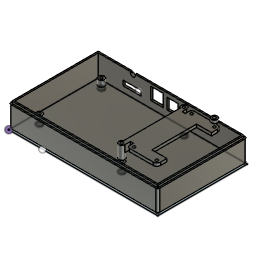
newSandProjectBox (Autodesk Fusion 360 design; units mm, degrees)
Autodesk Fusion 360 part; units mm, degrees
sketch "base " plane through (0, 0, 0) normal (0, 0, 1) x (1, 0, 0)
  line L0 (0, 0) -> (150, 0)
  line L1 (150, 0) -> (150, 90)
  line L2 (150, 90) -> (0, 90)
  line L3 (0, 90) -> (0, 0)
  circle A0 centre (10.5, 82.8) radius 3
  circle A1 centre (93.5, 82.8) radius 3
  circle A2 centre (93.5, 20.3) radius 3
  circle A3 centre (10.5, 20.3) radius 3
  point P0 (34, 0)
  point P1 (31.6409, 99.4995)
  dimension "d1" = 150
  dimension "d2" = 90
  dimension "d5" = 83
  dimension "d6" = 62.5
  dimension "d13" = 6
  dimension "d42" = 7.2
  dimension "d43" = 10.5
  constraint horizontal L0
  constraint vertical L1
  constraint horizontal L2
  constraint vertical L3
  constraint coincident L0.start L3.end
  measures "d1" distance of L0.start L0.end
  measures "d2" distance of L0.start L2.end
  measures "d13" diameter of A3
  measures "d42" distance of L2 A1.centre
  measures "d43" distance of L3 A3.centre
extrude "Extrude1" add sketch "base " along normal blind 25 contours L0 L1 L2 L3 | A0 | A1 | A2 | A3 makes body 1
shell "Shell1" thickness 3 removed faces 1 at (50, 60, 25) on bodies 1
sketch "back" plane through (0, 90, 0) normal (0, 1, 0) x (-1, 0, 0)
  line L0 (-150, 0) -> (0, 0)
  line L1 (0, 0) -> (0, 25)
  line L2 (0, 25) -> (-150, 25)
  line L3 (-150, 25) -> (-150, 0)
  circle A0 centre (-38, 24) radius 2.5
  line L4 (-28, 12.8) -> (-46, 12.8)
  line L5 (-56, 22.5) -> (-56, 10)
  line L6 (0, 25) -> (-123.61, 25)
  line L7 (-46, 12.8) -> (-46, 8.8)
  line L8 (-68.5, 22.5) -> (-56, 22.5)
  line L9 (-72.39, 21) -> (-72.39, 10)
  line L10 (-28, 8.8) -> (-28, 12.8)
  line L11 (-83.39, 10) -> (-83.39, 21)
  line L12 (-68.5, 10) -> (-68.5, 22.5)
  line L13 (-72.39, 10) -> (-83.39, 10)
  line L14 (-83.39, 21) -> (-72.39, 21)
  line L15 (-56, 10) -> (-68.5, 10)
  line L16 (-46, 8.8) -> (-28, 8.8)
  point P0 (0, 25)
  point P1 (-96, 0)
  point P2 (-96, 0)
  dimension "d25" = 12.5
  dimension "d26" = 12.5
  dimension "d27" = 11
  dimension "d28" = 11
  dimension "d34" = 18
  dimension "d35" = 4
  dimension "d37" = 5
  dimension "d107" = 28
  dimension "d108" = 56
  dimension "d109" = 72.39
  constraint horizontal L8
  constraint vertical L5
  constraint horizontal L15
  constraint vertical L12
  constraint horizontal L14
  constraint vertical L9
  constraint horizontal L13
  constraint vertical L11
  constraint coincident P2 P1
  constraint vertical L7
  constraint horizontal L16
  constraint vertical L10
  constraint perpendicular L4 L7
  measures "d25" distance of L8.start L5.start
  measures "d26" distance of L8.start L12.start
  measures "d27" distance of L11.end L9.start
  measures "d28" distance of L11.start L11.end
  measures "d34" distance of L4.end L4.start
  measures "d35" distance of L4.start L10.start
  measures "d37" diameter of A0
  measures "d107" distance of L1 L10
  measures "d108" distance of L1 L5
  measures "d109" distance of L1 L9
extrude "Extrude2" cut sketch "back" against normal blind 10 contours L2 A0 L6 | L4 L7 L10 L16 | L5 L8 L12 L15 | L9 L11 L13 L14 picked at (-38.7711, 24.4201) bodies 1
extrude "Extrude3" add sketch "base " along normal blind 9 contours A0 | A1 | A2 | A3 bodies 1
hole "Hole1" at (93.5, 20.3, 0) at (93.5, 82.8, 0) at (10.5, 20.3, 0) at (10.5, 82.8, 0) direction (0, 0, 1) diameter 2.529 depth 40 tip angle 118 bodies 1
thread "Thread1" "ISO Metric profile 3.0 M3x0.5 6H" major diameter 3.086 minor diameter 2.529 pitch 0.5 angle 60 resizes the face on face at (93.812, 84.0254, 3) on face at (9.2547, 83.0196, 3) on face at (10.563, 21.5629, 3) on face at (93.0088, 21.4652, 3) on bodies 1
ref_plane "WorkPlane1" through (75, 45, 33) normal (0, 0, 1) x (1, 0, 0)
sketch "pj shelf" plane through (0, 0, 33) normal (0, 0, 1) x (1, 0, 0)
  line L0 (125.7136, 84.4885) -> (102.4203, 84.4885)
  arc A0 (129.6079, 80.5942) -> (125.7136, 84.4885) centre (125.7136, 80.5942) ccw
  line L1 (99.6079, 81.6761) -> (99.6079, 21.7573)
  circle A1 centre (126.1079, 80.9885) radius 1.375
  circle A2 centre (126.1079, 22.9885) radius 3
  circle A3 centre (126.1079, 80.9885) radius 3
  circle A4 centre (103.1079, 80.9885) radius 1.375
  line L2 (129.6079, 23.2558) -> (129.6079, 80.5942)
  circle A5 centre (103.1079, 80.9885) radius 3
  arc A6 (125.8406, 19.4885) -> (129.6079, 23.2558) centre (125.8406, 23.2558) ccw
  arc A7 (99.6079, 21.7573) -> (101.8768, 19.4885) centre (101.8768, 21.7573) ccw
  arc A8 (102.4203, 84.4885) -> (99.6079, 81.6761) centre (102.4203, 81.6761) ccw
  circle A9 centre (103.1079, 22.9885) radius 3
  circle A10 centre (126.1079, 22.9885) radius 1.375
  circle A11 centre (103.1079, 22.9885) radius 1.375
  line L3 (101.8768, 19.4885) -> (125.8406, 19.4885)
  line L4 (114.6079, 74.481) -> (129.6079, 74.481)
  line L5 (129.6079, 29.481) -> (114.6079, 29.481)
  line L6 (114.6079, 29.481) -> (114.6079, 74.481)
  circle A12 centre (93.5, 20.3) radius 3
  circle A13 centre (93.5, 82.8) radius 3
  line L7 (90.5264, 20.3746) -> (90.5264, 20.6969)
  line L8 (96.4996, 20.5) -> (96.4996, 20.3497)
  line L9 (96.4996, 20.3497) -> (92.3791, 20.3497)
  line L10 (92.3791, 20.3497) -> (92.3791, 85.5827)
  line L11 (92.3791, 85.5827) -> (96.4996, 85.5827)
  line L12 (96.4996, 85.5827) -> (96.4996, 20.3497)
  line L13 (93.5, 20.3) -> (93.5, 82.8)
  line L14 (93.5, 25.983) -> (103.8671, 25.983)
  line L15 (103.8671, 25.983) -> (103.8671, 78.0861)
  line L16 (103.8671, 78.0861) -> (93.5, 78.0861)
  line L17 (93.5, 78.0861) -> (93.5, 25.983)
  line L18 (93.5, 30) -> (96.4996, 30)
  line L19 (93.5, 75) -> (99.6079, 75)
  point P0 (107.5942, 54.2702)
  dimension "d54" = 2.75
  dimension "d55" = 2.75
  dimension "d56" = 2.75
  dimension "d57" = 2.75
  dimension "d119" = 23
  dimension "d121" = 3.5
  dimension "d122" = 3.5
  dimension "d123" = 30
  dimension "d124" = 15
  dimension "d125" = 23
  dimension "d126" = 3.5
  dimension "d127" = 58
  dimension "d128" = 58
  dimension "d142" = 37.2288
  dimension "d146" = 65
  dimension "d147" = 3.5
  constraint concentric A1 A3
  constraint concentric A2 A10
  constraint concentric A9 A11
  constraint horizontal L4
  constraint horizontal L5
  constraint vertical L6
  constraint coincident A4.centre A5.centre
  constraint vertical L7
  constraint vertical L8
  constraint coincident A12 L7.end
  constraint coincident A12 L8.end
  constraint horizontal L9
  constraint vertical L10
  constraint horizontal L11
  constraint vertical L12
  constraint coincident A13 L10.end
  constraint coincident A12.centre L13.start
  constraint coincident A13.centre L13.end
  constraint horizontal L14
  constraint vertical L15
  constraint horizontal L16
  constraint vertical L17
  constraint coincident A5 L15.end
  constraint coincident L13 L14.start
  constraint coincident L13 L18.start
  constraint coincident L12 L18.end
  constraint perpendicular L1 L18
  constraint coincident L17 L19.start
  constraint coincident L1 L19.end
  constraint perpendicular L1 L19
  constraint horizontal L3
  constraint horizontal L0
  constraint tangent A7 L3
  constraint tangent L1 A7
  constraint tangent A6 L3
  constraint tangent L2 A6
  constraint tangent A0 L2
  constraint tangent L0 A0
  constraint tangent L0 A8
  constraint tangent L1 A8
  constraint coincident L2 L5.start
  constraint coincident L2 L4.end
  measures "d54" diameter of A1
  measures "d55" diameter of A4
  measures "d56" diameter of A10
  measures "d57" diameter of A11
  measures "d119" distance of A9.centre A2.centre
  measures "d121" distance of A2.centre L2
  measures "d122" distance of A1.centre L2
  measures "d123" distance of L1 L2
  measures "d124" distance of L1 L6
  measures "d125" horizontal distance of A4.centre A1.centre
  measures "d126" distance of A2.centre L3
  measures "d127" distance of A9.centre A4.centre
  measures "d128" distance of A2.centre A1.centre
  measures "d142" distance of L2 L10
  measures "d146" distance of L0 L3
  measures "d147" distance of A9.centre L3
extrude "Extrude4" add sketch "pj shelf" along normal blind 3 separate body contours L0 A0 L1 L2 A5 A6 A7 A8 A9 L3 L4 L5 L6 L14 L15 L16 | L1 A5 A9 L14 L15 L16 | L1 L12 L16 L19 | L1 L12 L14 L19 | A5 L16 | A5 L16 | A13 L12 L13 L16 | L12 L13 L16 L17 L19 | L12 L13 L17 L18 L19 | A13 L10 L11 | A12 A13 L10 L13 L17 | L12 L13 L14 L17 L18 | A12 L8 L12 L13 L14 | A9 L14 | A9 L14 | A13 L11 | A12 L9 L13 | A12 L9 L10 | A12 L9 L10 L13 | A2 | A3 makes body 2
extrude "Extrude6" add sketch "pj shelf" along normal blind 3 contours A13 L12 L13 L16 | L12 L13 L16 L17 L19 | L12 L13 L17 L18 L19 | A13 L10 L11 | L12 L13 L14 L17 L18 | A12 L8 L12 L13 L14 | A13 L11 | A13 L10 | A12 L9 L13 | A12 L9 L10 L13 bodies 2
extrude "Extrude7" add sketch "pj shelf" against normal blind 10 contours A13 L10 L11 | A13 L11 | A13 L10 | A12 L9 L13 | A12 L9 L10 | A12 L9 L10 L13 bodies 2
fillet "Fillet1" radius 2 8 edges at (150, 0, 12.5) (0, 0, 12.5) (150, 90, 12.5) (0, 90, 12.5) (0, 45, 0) (75, 90, 0) (75, 0, 0) (150, 45, 0) on bodies 1
chamfer "Chamfer1" distance 1 angle 45 12 edges at (77.89, 90, 10) (83.39, 90, 15.5) (77.89, 90, 21) (72.39, 90, 15.5) (68.5, 90, 16.25) (62.25, 90, 22.5) (56, 90, 16.25) (62.25, 90, 10) (37, 90, 8.8) (28, 90, 10.8) (37, 87, 12.8) (46, 90, 10.8) on bodies 1
sketch "rim of box" plane through (0, 0, 25) normal (0, 0, 1) x (-1, 0, 0)
  line L0 (-40.2913, -87) -> (-147, -87)
  line L1 (-147, -87) -> (-147, -3)
  line L2 (-147, -3) -> (-3, -3)
  line L3 (-3, -3) -> (-3, -87)
  arc A0 (-148, 0) -> (-150, -2) centre (-148, -2) ccw
  line L4 (-150, -2) -> (-150, -88)
  arc A1 (-150, -88) -> (-148, -90) centre (-148, -88) ccw
  line L5 (-148, -90) -> (-40.2913, -90)
  arc A2 (-2, -90) -> (0, -88) centre (-2, -88) ccw
  line L6 (0, -88) -> (0, -2)
  arc A3 (0, -2) -> (-2, 0) centre (-2, -2) ccw
  line L7 (-2, 0) -> (-148, 0)
  line L8 (-3, -87) -> (-35.7087, -87)
  line L9 (-35.7087, -90) -> (-2, -90)
  arc A4 (-2, -88.5) -> (-1.5, -88) centre (-2, -88) ccw
  line L10 (-1.5, -88) -> (-1.5, -2)
  arc A5 (-1.5, -2) -> (-2, -1.5) centre (-2, -2) ccw
  line L11 (-2, -1.5) -> (-148, -1.5)
  arc A6 (-148, -1.5) -> (-148.5, -2) centre (-148, -2) ccw
  line L12 (-148.5, -2) -> (-148.5, -88)
  arc A7 (-148.5, -88) -> (-148, -88.5) centre (-148, -88) ccw
  line L13 (-148, -88.5) -> (-40.2913, -88.5)
  line L14 (-40.2913, -90) -> (-35.7087, -90)
  line L15 (-35.7087, -77) -> (-40.2913, -77)
  line L16 (-40.2913, -88.5) -> (-2, -88.5)
  dimension "d92" = -1.5
  constraint coincident L5.end L14.start
  constraint coincident L9.start L14.end
  constraint coincident L8.end L15.start
  constraint coincident L0.start L15.end
  constraint tangent A4 L16
extrude "Extrude9" cut sketch "rim of box" against normal blind 2 bodies 1
move_body "Move1" bodies 2 to x (1, 0, 0) y (0, 1, 0) z (0, 0, 1) at (0, 0, -7)
extrude "Extrude11" add sketch "pj shelf" against normal blind 3 separate body contours A3 makes body 3
move_face "OffsetFaces1" offset -0.2 1 faces at (126.3467, 82.3426, 31) on bodies 3
hole "Hole6" at (93.5, 82.8, 33) at (93.5, 20.3, 33) direction (0, 0, -1) diameter 2.8016 depth 30 tip angle 118 bodies 2
extrude "Extrude12" add sketch "pj shelf" against normal blind 7 from surface at -4 contours L1 A5 A9 L14 L15 L16 | L1 L12 L16 L19 | L1 L12 L14 L19 | A13 L12 L13 L16 | L12 L13 L16 L17 L19 | L12 L13 L14 L17 L18 | A12 L8 L12 L13 L14 | A9 L14 picked at (103.0879, 25.9846) bodies 2
fillet "Fillet6" radius 2 1 edges at (93.5, 75, 24) on bodies 2
move_body "Move2" bodies 2 to x (1, 0, 0) y (0, 1, 0) z (0, 0, 1) at (0, 0, -4)
move_face "MoveFace1" to x (1, 0, 0) y (0, 1, 0) z (0, 0, 1) at (0, 0, -4) 1 faces at (124.1229, 78.7391, 31) on bodies 3
sketch "Sketch5" plane through (0, 0, 3) normal (0, 0, 1) x (-1, 0, 0)
  circle A0 centre (-93.5, -82.8) radius 3
  circle A1 centre (-10.5, -82.8) radius 3
  circle A2 centre (-10.5, -20.3) radius 3
  circle A3 centre (-93.5, -20.3) radius 3
  line L0 (-3, -87) -> (-3, -3)
  line L1 (-3, -3) -> (-147, -3)
  line L2 (-147, -3) -> (-147, -87)
  line L3 (-147, -87) -> (-3, -87)
move_body "Move3" [suppressed]
equation "d122 = d121"
equation "d125 = d119"
equation "d127 = d128"
equation "d147 = d126"
named bodies: "omnabad project base", "pi standoff", "pi shelf"
